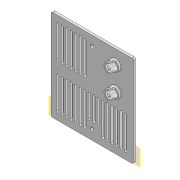
# Autodesk Inventor part: fechamento1
Saved by Autodesk Inventor 2020 (Build 240168000, 168)
## iProperties
Created: 2022-08-02
Part Number: fechamento1
Material: Genérico
Document SubType Name: Modeling
Designer: gabri
Density: 1 g/cm^3
Appearance: Padrão
Author: gabri
Autodesk Inventor part; units mm, degrees
ref_plane "YZ Plane" through (0, 0, 0) normal (1, 0, 0) x (0, 1, 0)
ref_plane "XZ Plane" through (0, 0, 0) normal (0, 1, 0) x (-1, 0, 0)
ref_plane "XY Plane" through (0, 0, 0) normal (0, 0, 1) x (1, 0, 0)
ref_plane "Plano de trabalho1" through (0, 0, 0) normal (0, 0, 1) x (1, 0, 0)
sketch "Esboço1" plane through (0, 0, 0) normal (0, 0, 1) x (1, 0, 0)
  arc A0 (62, 11) -> (61, 12) centre (61, 11) ccw
  line L0 (61, 12) -> (49, 12)
  arc A1 (49, 12) -> (48, 11) centre (49, 11) ccw
  line L1 (48, 1) -> (48, 11)
  arc A2 (47, 0) -> (48, 1) centre (47, 1) ccw
  line L2 (11, 0) -> (47, 0)
  arc A3 (10, 1) -> (11, 0) centre (11, 1) ccw
  line L3 (10, 1) -> (10, 9)
  line L4 (0, 9) -> (10, 9)
  line L5 (0, -8) -> (0, 9)
  line L6 (0, -8) -> (110, -8)
  line L7 (110, -8) -> (110, 9)
  line L8 (100, 9) -> (110, 9)
  line L9 (100, 1) -> (100, 9)
  arc A4 (99, 0) -> (100, 1) centre (99, 1) ccw
  line L10 (63, 0) -> (99, 0)
  arc A5 (62, 1) -> (63, 0) centre (63, 1) ccw
  line L11 (62, 11) -> (62, 1)
  circle A6 centre (55, 6) radius 2.25
  arc A7 (48, 96) -> (49, 95) centre (49, 96) ccw
  line L12 (61, 95) -> (49, 95)
  arc A8 (61, 95) -> (62, 96) centre (61, 96) ccw
  line L13 (62, 106) -> (62, 96)
  arc A9 (63, 107) -> (62, 106) centre (63, 106) ccw
  line L14 (63, 107) -> (99.2679, 107)
  spline S0 degree 3 poles (101, 106) (100.7229, 106.2771) (100.3848, 106.6039) (99.8153, 106.9104) (99.5228, 107) (99.2679, 107) knots 0 0 0 0 0.605913 0.605913 1 1 1 1
  line L15 (101, 98) -> (101, 106)
  line L16 (110, 98) -> (101, 98)
  line L17 (110, 115) -> (110, 98)
  line L18 (0, 115) -> (110, 115)
  line L19 (0, 115) -> (0, 98)
  line L20 (10, 98) -> (0, 98)
  line L21 (10, 106) -> (10, 98)
  arc A10 (11, 107) -> (10, 106) centre (11, 106) ccw
  line L22 (11, 107) -> (47, 107)
  arc A11 (48, 106) -> (47, 107) centre (47, 106) ccw
  line L23 (48, 96) -> (48, 106)
  circle A12 centre (55, 101) radius 2.25
  line L24 (109.5, 114) -> (0.5, 114)
  line L25 (0.5, 114) -> (0.5, -7)
  line L26 (0.5, -7) -> (109.5, -7)
  line L27 (109.5, -7) -> (109.5, 114)
  line L28 (55, 101.5) -> (55, 100.5)
  line L29 (55, 101.5) -> (55, 100.5) construction
  line L30 (52.75, 101.5) -> (52.75, 100.5)
  line L31 (57.25, 100.5) -> (57.25, 101.5)
  arc A13 (57.25, 101.5) -> (52.75, 101.5) centre (55, 101.5) ccw
  arc A14 (52.75, 100.5) -> (57.25, 100.5) centre (55, 100.5) ccw
  circle A15 centre (55, 6) radius 0.25
  line L32 (55, 6.25) -> (55, 5.75) construction
  line L33 (52.75, 6.25) -> (52.75, 5.75)
  line L34 (57.25, 5.75) -> (57.25, 6.25)
  arc A16 (57.25, 6.25) -> (52.75, 6.25) centre (55, 6.25) ccw
  arc A17 (52.75, 5.75) -> (57.25, 5.75) centre (55, 5.75) ccw
  circle A18 centre (86.5, 96) radius 5
  circle A19 centre (86.5, 65) radius 5
  line L35 (45.1388, 104) -> (45.1388, 62) construction
  line L36 (46.7388, 104) -> (46.7388, 62)
  line L37 (43.5388, 62) -> (43.5388, 104)
  arc A20 (46.7388, 104) -> (43.5388, 104) centre (45.1388, 104) ccw
  arc A21 (43.5388, 62) -> (46.7388, 62) centre (45.1388, 62) ccw
  line L38 (45.1388, 45) -> (45.1388, 3) construction
  line L39 (46.7388, 45) -> (46.7388, 3)
  line L40 (43.5388, 3) -> (43.5388, 45)
  arc A22 (46.7388, 45) -> (43.5388, 45) centre (45.1388, 45) ccw
  arc A23 (43.5388, 3) -> (46.7388, 3) centre (45.1388, 3) ccw
  arc A24 (37.5388, 62) -> (40.7388, 62) centre (39.1388, 62) ccw
  arc A25 (40.7388, 45) -> (37.5388, 45) centre (39.1388, 45) ccw
  line L41 (40.7388, 104) -> (40.7388, 62)
  line L42 (39.1388, 104) -> (39.1388, 62) construction
  line L43 (37.5388, 62) -> (37.5388, 104)
  arc A26 (40.7388, 104) -> (37.5388, 104) centre (39.1388, 104) ccw
  line L44 (40.7388, 45) -> (40.7388, 3)
  line L45 (39.1388, 45) -> (39.1388, 3) construction
  line L46 (37.5388, 3) -> (37.5388, 45)
  arc A27 (37.5388, 3) -> (40.7388, 3) centre (39.1388, 3) ccw
  arc A28 (31.5388, 62) -> (34.7388, 62) centre (33.1388, 62) ccw
  arc A29 (34.7388, 45) -> (31.5388, 45) centre (33.1388, 45) ccw
  line L47 (34.7388, 104) -> (34.7388, 62)
  line L48 (33.1388, 104) -> (33.1388, 62) construction
  line L49 (31.5388, 62) -> (31.5388, 104)
  arc A30 (34.7388, 104) -> (31.5388, 104) centre (33.1388, 104) ccw
  line L50 (34.7388, 45) -> (34.7388, 3)
  line L51 (33.1388, 45) -> (33.1388, 3) construction
  line L52 (31.5388, 3) -> (31.5388, 45)
  arc A31 (31.5388, 3) -> (34.7388, 3) centre (33.1388, 3) ccw
  arc A32 (25.5388, 62) -> (28.7388, 62) centre (27.1388, 62) ccw
  arc A33 (28.7388, 45) -> (25.5388, 45) centre (27.1388, 45) ccw
  line L53 (28.7388, 104) -> (28.7388, 62)
  line L54 (27.1388, 104) -> (27.1388, 62) construction
  line L55 (25.5388, 62) -> (25.5388, 104)
  arc A34 (28.7388, 104) -> (25.5388, 104) centre (27.1388, 104) ccw
  line L56 (28.7388, 45) -> (28.7388, 3)
  line L57 (27.1388, 45) -> (27.1388, 3) construction
  line L58 (25.5388, 3) -> (25.5388, 45)
  arc A35 (25.5388, 3) -> (28.7388, 3) centre (27.1388, 3) ccw
  arc A36 (19.5388, 62) -> (22.7388, 62) centre (21.1388, 62) ccw
  arc A37 (22.7388, 45) -> (19.5388, 45) centre (21.1388, 45) ccw
  line L59 (22.7388, 104) -> (22.7388, 62)
  line L60 (21.1388, 104) -> (21.1388, 62) construction
  line L61 (19.5388, 62) -> (19.5388, 104)
  arc A38 (22.7388, 104) -> (19.5388, 104) centre (21.1388, 104) ccw
  line L62 (22.7388, 45) -> (22.7388, 3)
  line L63 (21.1388, 45) -> (21.1388, 3) construction
  line L64 (19.5388, 3) -> (19.5388, 45)
  arc A39 (19.5388, 3) -> (22.7388, 3) centre (21.1388, 3) ccw
  arc A40 (13.5388, 62) -> (16.7388, 62) centre (15.1388, 62) ccw
  arc A41 (16.7388, 45) -> (13.5388, 45) centre (15.1388, 45) ccw
  line L65 (16.7388, 104) -> (16.7388, 62)
  line L66 (15.1388, 104) -> (15.1388, 62) construction
  line L67 (13.5388, 62) -> (13.5388, 104)
  arc A42 (16.7388, 104) -> (13.5388, 104) centre (15.1388, 104) ccw
  line L68 (16.7388, 45) -> (16.7388, 3)
  line L69 (15.1388, 45) -> (15.1388, 3) construction
  line L70 (13.5388, 3) -> (13.5388, 45)
  arc A43 (13.5388, 3) -> (16.7388, 3) centre (15.1388, 3) ccw
  arc A44 (7.5388, 62) -> (10.7388, 62) centre (9.1388, 62) ccw
  arc A45 (10.7388, 45) -> (7.5388, 45) centre (9.1388, 45) ccw
  line L71 (10.7388, 104) -> (10.7388, 62)
  line L72 (9.1388, 104) -> (9.1388, 62) construction
  line L73 (7.5388, 62) -> (7.5388, 104)
  arc A46 (10.7388, 104) -> (7.5388, 104) centre (9.1388, 104) ccw
  line L74 (10.7388, 45) -> (10.7388, 3)
  line L75 (9.1388, 45) -> (9.1388, 3) construction
  line L76 (7.5388, 3) -> (7.5388, 45)
  arc A47 (7.5388, 3) -> (10.7388, 3) centre (9.1388, 3) ccw
  line L77 (51.1388, 45) -> (51.1388, 15.5537) construction
  line L78 (49.5388, 45) -> (49.5388, 15.5537)
  line L79 (52.7388, 15.5537) -> (52.7388, 45)
  arc A48 (52.7388, 45) -> (49.5388, 45) centre (51.1388, 45) ccw
  arc A49 (49.5388, 15.5537) -> (52.7388, 15.5537) centre (51.1388, 15.5537) ccw
  line L80 (55.5388, 45) -> (55.5388, 15.5537)
  line L81 (57.1388, 45) -> (57.1388, 15.5537) construction
  arc A50 (55.5388, 15.5537) -> (58.7388, 15.5537) centre (57.1388, 15.5537) ccw
  line L82 (58.7388, 15.5537) -> (58.7388, 45)
  arc A51 (58.7388, 45) -> (55.5388, 45) centre (57.1388, 45) ccw
  line L83 (61.5388, 45) -> (61.5388, 15.5537)
  line L84 (63.1388, 45) -> (63.1388, 15.5537) construction
  arc A52 (61.5388, 15.5537) -> (64.7388, 15.5537) centre (63.1388, 15.5537) ccw
  line L85 (64.7388, 15.5537) -> (64.7388, 45)
  arc A53 (64.7388, 45) -> (61.5388, 45) centre (63.1388, 45) ccw
  line L86 (69.1388, 45) -> (69.1388, 3) construction
  line L87 (67.5388, 45) -> (67.5388, 3)
  line L88 (70.7388, 3) -> (70.7388, 45)
  arc A54 (70.7388, 45) -> (67.5388, 45) centre (69.1388, 45) ccw
  arc A55 (67.5388, 3) -> (70.7388, 3) centre (69.1388, 3) ccw
  arc A56 (76.7388, 45) -> (73.5388, 45) centre (75.1388, 45) ccw
  line L89 (73.5388, 45) -> (73.5388, 3)
  line L90 (75.1388, 45) -> (75.1388, 3) construction
  arc A57 (73.5388, 3) -> (76.7388, 3) centre (75.1388, 3) ccw
  line L91 (76.7388, 3) -> (76.7388, 45)
  arc A58 (82.7388, 45) -> (79.5388, 45) centre (81.1388, 45) ccw
  line L92 (79.5388, 45) -> (79.5388, 3)
  line L93 (81.1388, 45) -> (81.1388, 3) construction
  arc A59 (79.5388, 3) -> (82.7388, 3) centre (81.1388, 3) ccw
  line L94 (82.7388, 3) -> (82.7388, 45)
  arc A60 (88.7388, 45) -> (85.5388, 45) centre (87.1388, 45) ccw
  line L95 (85.5388, 45) -> (85.5388, 3)
  line L96 (87.1388, 45) -> (87.1388, 3) construction
  arc A61 (85.5388, 3) -> (88.7388, 3) centre (87.1388, 3) ccw
  line L97 (88.7388, 3) -> (88.7388, 45)
  arc A62 (94.7388, 45) -> (91.5388, 45) centre (93.1388, 45) ccw
  line L98 (91.5388, 45) -> (91.5388, 3)
  line L99 (93.1388, 45) -> (93.1388, 3) construction
  arc A63 (91.5388, 3) -> (94.7388, 3) centre (93.1388, 3) ccw
  line L100 (94.7388, 3) -> (94.7388, 45)
  line L101 (97.5388, 45) -> (97.5388, 3)
  line L102 (99.1388, 45) -> (99.1388, 3) construction
  line L103 (100.7388, 3) -> (100.7388, 45)
  arc A64 (100.7388, 45) -> (97.5388, 45) centre (99.1388, 45) ccw
  arc A65 (97.5388, 3) -> (100.7388, 3) centre (99.1388, 3) ccw
  point P0 (0, 0)
  point P1 (55, 101)
  point P2 (45.1388, 83)
  point P3 (45.1388, 24)
  point P4 (42, 106)
  point P5 (39.1388, 83)
  point P6 (39.1388, 24)
  point P7 (36, 106)
  point P8 (33.1388, 83)
  point P9 (33.1388, 24)
  point P10 (30, 106)
  point P11 (27.1388, 83)
  point P12 (27.1388, 24)
  point P13 (24, 106)
  point P14 (21.1388, 83)
  point P15 (21.1388, 24)
  point P16 (18, 106)
  point P17 (15.1388, 83)
  point P18 (15.1388, 24)
  point P19 (12, 106)
  point P20 (9.1388, 83)
  point P21 (9.1388, 24)
  point P22 (51.1388, 30.2768)
  point P23 (57.1388, 30.2768)
  point P24 (63.1388, 30.2768)
  point P25 (69.1388, 24)
  point P26 (75.1388, 24)
  point P27 (81.1388, 24)
  point P28 (87.1388, 24)
  point P29 (93.1388, 24)
  point P30 (99.1388, 24)
  dimension "d0" = 0.5
  dimension "d1" = 0.5
  dimension "d2" = 1
  dimension "d3" = 1
  dimension "d4" = 0.5
  dimension "d5" = 0.5
  dimension "d6" = 4.5
  dimension "d7" = 0.5
  dimension "d8" = 4.5
  dimension "d9" = 10
  dimension "d10" = 10
  dimension "d11" = 18
  dimension "d12" = 23
  dimension "d13" = 23
  dimension "d14" = 31
  dimension "d15" = 42
  dimension "d16" = 42
  dimension "d17" = 31
  dimension "d18" = 31
  dimension "d19" = 3.2
  dimension "d20" = 3.2
  dimension "d23" = 6
  dimension "d30" = 3.2
  dimension "d31" = 6
  dimension "d34" = 6
  dimension "d39" = 3.2
  dimension "d40" = 6
  dimension "d43" = 6
  dimension "d50" = 6
  constraints: 210 end point, 102 point on circle, 53 centre point, 24 tangent, 14 point on line, 9 equal length, 6 midpoint, 5 horizontal, 5 vertical, 1 coincident, 1 perpendicular, 234 other
  measures "d0" distance between parallel lines of L17 L27
  measures "d1" distance from line of L19.end L25
  measures "d2" distance between parallel lines of L18 L24
  measures "d3" distance between parallel lines of L6 L26
  measures "d4" distance of L28.start A12.centre
  measures "d5" distance of L28.end A12.centre
  measures "d6" diameter of A14
  measures "d7" diameter of A15
  measures "d8" diameter of A17
  measures "d9" diameter of A18
  measures "d10" diameter of A19
  measures "d11" distance from line of L24 A18.centre
  measures "d12" distance from line of L27 A18.centre
  measures "d13" distance from line of L27 A19.centre
  measures "d14" distance of A19.centre A18.centre
  measures "d15" distance of L35.start L35.end
  measures "d16" distance of L38.start L38.end
  measures "d17" distance from line of L24 point (45.139, 83)
  measures "d18" distance from line of L26 point (45.139, 24)
  measures "d19" distance between parallel lines of L37 L36
  measures "d20" distance between parallel lines of L40 L39
  measures "d23" distance of L23.end point (42, 106)
  measures "d30" diameter of A49
  measures "d31" distance between parallel lines of L40 L78
  measures "d34" distance of L77.start L81.start
  measures "d39" diameter of A55
  measures "d40" horizontal distance of point (63.139, 30.277) point (69.139, 24)
  measures "d43" distance of L86.start L90.start
  measures "d50" distance of L98.start L101.start
extrude "Extrusão1" add sketch "Esboço1" along normal blind 3 contours L11 A5 L10 A4 L9 A65 L103 L8 L27 L26 L25 L4 L76 A47 L3 A3 L2 A2 L1 A1 L0 A0 | A0 L0 A1 L1 A2 L2 A3 L3 A47 L74 A45 L76 L4 L25 L20 L73 A44 L71 A46 L21 A10 L22 A11 L23 A7 L12 A8 L13 A9 L14 S0 L15 L16 L27 L8 L103 A64 L101 A65 L9 A4 L10 A5 L11 | L16 L15 S0 L14 A9 L13 A8 L12 A7 L23 A11 L22 A10 L21 A46 L73 L20 L25 L24 L27
sketch "Esboço2" plane through (0, 0, 3) normal (0, 0, 1) x (1, 0, 0)
  circle A0 centre (86.5, 96) radius 5 projected
  circle A1 centre (86.5, 96) radius 7
  circle A2 centre (86.5, 65) radius 5 projected
  circle A3 centre (86.5, 65) radius 7
  point P0 (0, 0)
  dimension "d55" = 14
  dimension "d56" = 14
  constraints: 2 centre point, 2 coincident
  measures "d55" diameter of A1
  measures "d56" diameter of A3
extrude "Extrusão2" add sketch "Esboço2" along normal blind 3
fillet "Arredondamento1" radius 0.5 2 edges at (79.5, 96, 3) (79.5, 65, 3)
sketch "Esboço3" plane through (86.5, 96, 6) normal (0, 0, 1) x (1, 0, 0)
  circle A0 centre (0, 0) radius 7 projected
  circle A1 centre (0, 0) radius 5 projected
  circle A2 centre (0, -31) radius 7 projected
  circle A3 centre (0, -31) radius 5 projected
  circle A4 centre (0, 0) radius 7 projected
  line L0 (0, 7) -> (0, -7)
  circle A5 centre (0, -31) radius 7 projected
  line L1 (0, -24) -> (0, -38)
  point P0 (-86.5, -96)
  point P1 (0, -36)
  point P2 (0, -26)
  point P3 (0, -24)
  point P4 (0, -7)
  point P5 (0, -5)
  point P6 (0, 5)
  point P7 (0, 7)
  constraints: 4 end point, 4 point on circle, 2 point on line, 1 vertical
extrude "Extrusão3" add sketch "Esboço3" along normal blind 6 contours L0 A1 A0 | L1 A3 A2 picked at (-0.9573, -6.2171) picked at (-0.9573, -37.2171)
sketch "Esboço4" plane through (0.5, 114, 0) normal (0, 1, 0) x (1, 0, 0)
  circle A0 centre (82.6921, -8.9568) radius 1.5
  point P0 (-0.5, 0)
  dimension "d62" = 3
  constraints: 1 centre point
  measures "d62" diameter of A0
extrude "Extrusão4" cut sketch "Esboço4" against normal blind 100
fillet "Arredondamento2" radius 2 12 edges at (86.5, 102, 12) (86.5, 102, 6) (86.5, 90, 6) (86.5, 90, 12) (86.5, 71, 6) (86.5, 71, 12) (86.5, 59, 12) (86.5, 59, 6) (109.5, -7, 1.5) (0.5, -7, 1.5) (0.5, 114, 1.5) (109.5, 114, 1.5)
equation "\"d13\" = d12"
equation "\"d16\" = d15"
equation "\"d18\" = d17"
equation "\"d20\" = d19"
